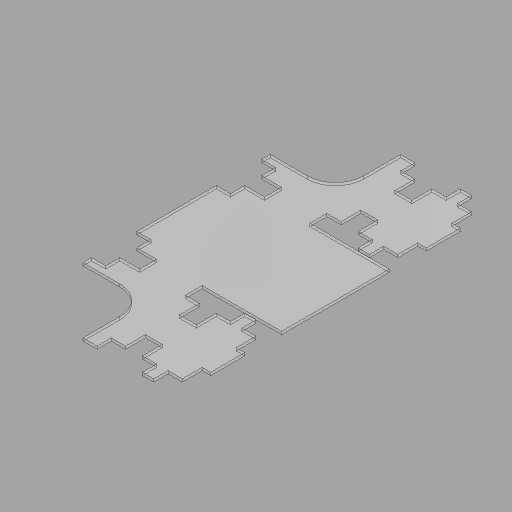
# Autodesk Inventor part: 2024-100-006-Electrical-Plate
Saved by Autodesk Inventor 2024.2 (Build 282272000, 272)
## iProperties
Created: 2024-02-14
Part Number: 2024-100-006-Electrical-Plate
Material: Polycarbonate, Clear
Document SubType Name: Modeling
Designer: rohan
Density: 1.2 g/cm^3
Appearance: Polycarbonate - Clear
Author: rohan
Autodesk Inventor part; units mm, degrees
ref_plane "YZ Plane" through (0, 0, 0) normal (1, 0, 0) x (0, 1, 0)
ref_plane "XZ Plane" through (0, 0, 0) normal (0, 1, 0) x (-1, 0, 0)
ref_plane "XY Plane" through (0, 0, 0) normal (0, 0, 1) x (1, 0, 0)
sketch "Sketch1" plane through (0, 0, 0) normal (0, 1, 0) x (-1, 0, 0)
  line L0 (355.6, 355.6) -> (-355.6, 355.6)
  line L1 (-355.6, 355.6) -> (-355.6, -355.6)
  line L2 (-355.6, -355.6) -> (355.6, -355.6)
  line L3 (355.6, -355.6) -> (355.6, 355.6)
  line L4 (355.6, 355.6) -> (-355.6, -355.6) construction
  line L5 (-355.6, 355.6) -> (355.6, -355.6) construction
  point P0 (0, 0)
  dimension "d0" = 711.2
  dimension "d1" = 711.2
  constraints: 12 end point, 2 midpoint, 2 parallel, 1 horizontal, 1 perpendicular
  measures "d0" distance of L2.end L1.end
  measures "d1" distance of L1.end L0.end
extrude "Extrusion1" add sketch "Sketch1" along normal blind 6.35
sketch "Sketch2" plane through (0, 6.35, 0) normal (0, 1, 0) x (1, 0, 0)
  line L0 (355.6, -355.6) -> (355.6, 355.6) projected
  line L1 (355.6, 355.6) -> (-355.6, 355.6) projected
  line L2 (-355.6, 355.6) -> (-355.6, -355.6) projected
  line L3 (-355.6, -355.6) -> (355.6, -355.6) projected
  line L4 (-355.6, -355.6) -> (-279.4, -355.6)
  line L5 (-279.4, -355.6) -> (-279.4, -323.85)
  line L6 (-279.4, -323.85) -> (-323.85, -323.85)
  line L7 (-323.85, -323.85) -> (-323.85, -279.4)
  line L8 (-323.85, -279.4) -> (-355.6, -279.4)
  line L9 (-355.6, 355.6) -> (-355.6, -355.6) projected
  line L10 (-355.6, -279.4) -> (-355.6, -355.6)
  line L11 (-424.5174, 0) -> (433.8456, 0) construction
  line L12 (0, -429.639) -> (0, 434.6438) construction
  line L13 (-355.6, -355.6) -> (-355.6, 355.6)
  line L14 (-355.6, 355.6) -> (355.6, 355.6)
  line L15 (-279.4, 355.6) -> (-279.4, 323.85)
  line L16 (-279.4, 323.85) -> (-323.85, 323.85)
  line L17 (-323.85, 323.85) -> (-323.85, 279.4)
  line L18 (-323.85, 279.4) -> (-355.6, 279.4)
  line L19 (355.6, 355.6) -> (355.6, -355.6)
  line L20 (355.6, -355.6) -> (279.4, -355.6)
  line L21 (279.4, -355.6) -> (279.4, -323.85)
  line L22 (279.4, -323.85) -> (323.85, -323.85)
  line L23 (323.85, -323.85) -> (323.85, -279.4)
  line L24 (323.85, -279.4) -> (355.6, -279.4)
  line L25 (355.6, 355.6) -> (355.6, -355.6)
  line L26 (355.6, -279.4) -> (355.6, -355.6)
  line L27 (323.85, 279.4) -> (355.6, 279.4)
  line L28 (279.4, 355.6) -> (279.4, 323.85)
  line L29 (279.4, 323.85) -> (323.85, 323.85)
  line L30 (323.85, 323.85) -> (323.85, 279.4)
  line L31 (355.6, -355.6) -> (355.6, 355.6)
  point P0 (0, 0)
  dimension "d4" = 76.2
  dimension "d5" = 31.75
  dimension "d6" = 44.45
  dimension "d7" = 44.45
  constraints: 54 end point, 21 symmetric about line, 6 point on line, 3 perpendicular, 2 vertical, 1 collinear, 1 horizontal
  measures "d4" distance of L2.end L4.end
  measures "d5" distance of L4.end L5.end
  measures "d6" distance of L5.end L6.end
  measures "d7" distance of L6.end L7.end
extrude "Extrusion2" cut sketch "Sketch2" against normal blind 6.35 contours L3 L21 L22 L23 L24 L0 | L27 L30 L29 L28 L1 L0 | L3 L2 L8 L7 L6 L5 | L15 L16 L17 L18 L2 L1
sketch "Sketch3" plane through (0, 6.35, 0) normal (0, 1, 0) x (1, 0, 0)
  line L0 (355.6, 279.4) -> (323.85, 279.4) projected
  line L1 (323.85, 279.4) -> (323.85, 323.85) projected
  line L2 (323.85, 323.85) -> (279.4, 323.85) projected
  line L3 (279.4, 323.85) -> (279.4, 355.6) projected
  line L4 (279.4, 355.6) -> (-279.4, 355.6) projected
  line L5 (-279.4, 355.6) -> (-279.4, 323.85) projected
  line L6 (-279.4, 323.85) -> (-323.85, 323.85) projected
  line L7 (-323.85, 323.85) -> (-323.85, 279.4) projected
  line L8 (-323.85, 279.4) -> (-355.6, 279.4) projected
  line L9 (-355.6, 279.4) -> (-355.6, -279.4) projected
  line L10 (-355.6, -279.4) -> (-323.85, -279.4) projected
  line L11 (-323.85, -279.4) -> (-323.85, -323.85) projected
  line L12 (-323.85, -323.85) -> (-279.4, -323.85) projected
  line L13 (-279.4, -323.85) -> (-279.4, -355.6) projected
  line L14 (-279.4, -355.6) -> (279.4, -355.6) projected
  line L15 (279.4, -355.6) -> (279.4, -323.85) projected
  line L16 (279.4, -323.85) -> (323.85, -323.85) projected
  line L17 (323.85, -323.85) -> (323.85, -279.4) projected
  line L18 (323.85, -279.4) -> (355.6, -279.4) projected
  line L19 (355.6, -279.4) -> (355.6, 279.4) projected
  line L20 (-279.4, -355.6) -> (-355.6, -355.6)
  line L21 (-355.6, -355.6) -> (-355.6, -279.4)
  line L22 (-355.6, -355.6) -> (-355.6, -190.5)
  line L23 (-355.6, 279.4) -> (-355.6, -279.4) projected
  line L24 (-355.6, -190.5) -> (-323.85, -190.5)
  line L25 (-323.85, -190.5) -> (-323.85, -158.75)
  line L26 (-323.85, -158.75) -> (-279.4, -158.75)
  line L27 (-279.4, -158.75) -> (-279.4, -120.65)
  line L28 (-279.4, -120.65) -> (-323.85, -120.65)
  line L29 (-323.85, -120.65) -> (-323.85, -88.9)
  line L30 (-323.85, -88.9) -> (-355.6, -88.9)
  line L31 (-355.6, -88.9) -> (-355.6, -190.5)
  line L32 (-429.9144, 0) -> (459.921, 0) construction
  line L33 (-355.6, -279.4) -> (-355.6, 279.4)
  line L34 (-355.6, 190.5) -> (-323.85, 190.5)
  line L35 (-323.85, 190.5) -> (-323.85, 158.75)
  line L36 (-323.85, 158.75) -> (-279.4, 158.75)
  line L37 (-279.4, 158.75) -> (-279.4, 120.65)
  line L38 (-279.4, 120.65) -> (-323.85, 120.65)
  line L39 (-323.85, 120.65) -> (-323.85, 88.9)
  line L40 (-323.85, 88.9) -> (-355.6, 88.9)
  point P0 (0, 0)
  dimension "d10" = 165.1
  dimension "d11" = 31.75
  dimension "d12" = 31.75
  dimension "d13" = 44.45
  dimension "d14" = 38.1
  dimension "d15" = 31.75
  constraints: 40 end point, 10 symmetric about line, 5 perpendicular, 4 horizontal, 2 point on line, 1 collinear, 1 vertical
  measures "d10" distance of L20.end L22.end
  measures "d11" distance of L22.end L24.end
  measures "d12" distance of L24.end L25.end
  measures "d13" distance of L25.end L26.end
  measures "d14" distance of L26.end L27.end
  measures "d15" distance of L28.end L29.end
extrude "Extrusion3" cut sketch "Sketch3" against normal blind 6.35 contours L9 L30 L29 L28 L27 L26 L25 L24 | L34 L35 L36 L37 L38 L39 L40 L9
sketch "Sketch4" plane through (0, 6.35, 0) normal (0, 1, 0) x (1, 0, 0)
  line L0 (-323.85, 88.9) -> (-355.6, 88.9) projected
  line L1 (-355.6, 88.9) -> (-355.6, -88.9) projected
  line L2 (-355.6, -88.9) -> (-323.85, -88.9) projected
  line L3 (-323.85, -88.9) -> (-323.85, -120.65) projected
  line L4 (-323.85, -120.65) -> (-279.4, -120.65) projected
  line L5 (-279.4, -120.65) -> (-279.4, -158.75) projected
  line L6 (-279.4, -158.75) -> (-323.85, -158.75) projected
  line L7 (-323.85, -158.75) -> (-323.85, -190.5) projected
  line L8 (-323.85, -190.5) -> (-355.6, -190.5) projected
  line L9 (-355.6, -190.5) -> (-355.6, -279.4) projected
  line L10 (-355.6, -279.4) -> (-323.85, -279.4) projected
  line L11 (-323.85, -279.4) -> (-323.85, -323.85) projected
  line L12 (-323.85, -323.85) -> (-279.4, -323.85) projected
  line L13 (-279.4, -323.85) -> (-279.4, -355.6) projected
  line L14 (-279.4, -355.6) -> (279.4, -355.6) projected
  line L15 (279.4, -355.6) -> (279.4, -323.85) projected
  line L16 (279.4, -323.85) -> (323.85, -323.85) projected
  line L17 (323.85, -323.85) -> (323.85, -279.4) projected
  line L18 (323.85, -279.4) -> (355.6, -279.4) projected
  line L19 (355.6, -279.4) -> (355.6, 279.4) projected
  line L20 (355.6, 279.4) -> (323.85, 279.4) projected
  line L21 (323.85, 279.4) -> (323.85, 323.85) projected
  line L22 (323.85, 323.85) -> (279.4, 323.85) projected
  line L23 (279.4, 323.85) -> (279.4, 355.6) projected
  line L24 (279.4, 355.6) -> (-279.4, 355.6) projected
  line L25 (-279.4, 355.6) -> (-279.4, 323.85) projected
  line L26 (-279.4, 323.85) -> (-323.85, 323.85) projected
  line L27 (-323.85, 323.85) -> (-323.85, 279.4) projected
  line L28 (-323.85, 279.4) -> (-355.6, 279.4) projected
  line L29 (-355.6, 279.4) -> (-355.6, 190.5) projected
  line L30 (-355.6, 190.5) -> (-323.85, 190.5) projected
  line L31 (-323.85, 190.5) -> (-323.85, 158.75) projected
  line L32 (-323.85, 158.75) -> (-279.4, 158.75) projected
  line L33 (-279.4, 158.75) -> (-279.4, 120.65) projected
  line L34 (-279.4, 120.65) -> (-323.85, 120.65) projected
  line L35 (-323.85, 120.65) -> (-323.85, 88.9) projected
  line L36 (-279.4, -355.6) -> (-355.6, -355.6)
  line L37 (-355.6, -355.6) -> (-209.55, -355.6)
  line L38 (-209.55, -355.6) -> (-209.55, -273.05)
  line L39 (-273.05, -209.55) -> (-355.6, -209.55)
  line L40 (-355.6, -355.6) -> (-355.6, -209.55)
  arc A0 (-209.55, -273.05) -> (-273.05, -209.55) centre (-273.05, -273.05) ccw
  line L41 (-440.4629, 0) -> (-405.206, 0)
  line L42 (-355.6, 190.5) -> (-355.6, 279.4)
  line L43 (-355.6, 355.6) -> (-209.55, 355.6)
  line L44 (-209.55, 355.6) -> (-209.55, 273.05)
  line L45 (-273.05, 209.55) -> (-355.6, 209.55)
  line L46 (-355.6, 355.6) -> (-355.6, 209.55)
  arc A1 (-273.05, 209.55) -> (-209.55, 273.05) centre (-273.05, 273.05) ccw
  line L47 (0, -524.0203) -> (0, -477.0111)
  line L48 (323.85, 88.9) -> (355.6, 88.9)
  line L49 (355.6, 88.9) -> (355.6, -88.9)
  line L50 (355.6, -88.9) -> (323.85, -88.9)
  line L51 (323.85, -88.9) -> (323.85, -120.65)
  line L52 (323.85, -120.65) -> (279.4, -120.65)
  line L53 (279.4, -120.65) -> (279.4, -158.75)
  line L54 (279.4, -158.75) -> (323.85, -158.75)
  line L55 (323.85, -158.75) -> (323.85, -190.5)
  line L56 (323.85, -190.5) -> (355.6, -190.5)
  line L57 (355.6, -190.5) -> (355.6, -279.4)
  line L58 (355.6, -279.4) -> (323.85, -279.4)
  line L59 (323.85, -279.4) -> (323.85, -323.85)
  line L60 (323.85, -323.85) -> (279.4, -323.85)
  line L61 (279.4, -323.85) -> (279.4, -355.6)
  line L62 (279.4, 355.6) -> (279.4, 323.85)
  line L63 (279.4, 323.85) -> (323.85, 323.85)
  line L64 (323.85, 323.85) -> (323.85, 279.4)
  line L65 (323.85, 279.4) -> (355.6, 279.4)
  line L66 (355.6, 279.4) -> (355.6, 190.5)
  line L67 (355.6, 190.5) -> (323.85, 190.5)
  line L68 (323.85, 190.5) -> (323.85, 158.75)
  line L69 (323.85, 158.75) -> (279.4, 158.75)
  line L70 (279.4, 158.75) -> (279.4, 120.65)
  line L71 (279.4, 120.65) -> (323.85, 120.65)
  line L72 (323.85, 120.65) -> (323.85, 88.9)
  line L73 (279.4, -355.6) -> (355.6, -355.6)
  line L74 (355.6, -355.6) -> (209.55, -355.6)
  line L75 (209.55, -355.6) -> (209.55, -273.05)
  line L76 (273.05, -209.55) -> (355.6, -209.55)
  line L77 (355.6, -355.6) -> (355.6, -209.55)
  arc A2 (273.05, -209.55) -> (209.55, -273.05) centre (273.05, -273.05) ccw
  line L78 (273.05, 209.55) -> (355.6, 209.55)
  arc A3 (209.55, 273.05) -> (273.05, 209.55) centre (273.05, 273.05) ccw
  line L79 (355.6, 190.5) -> (355.6, 279.4)
  line L80 (355.6, 355.6) -> (355.6, 209.55)
  line L81 (355.6, 355.6) -> (209.55, 355.6)
  line L82 (209.55, 355.6) -> (209.55, 273.05)
  point P0 (0, 0)
  point P1 (-209.55, -209.55)
  point P2 (209.55, -209.55)
  point P3 (-209.55, 355.6)
  point P4 (209.55, 355.6)
  point P5 (209.55, -355.6)
  dimension "d18" = 146.05
  dimension "d19" = 146.05
  dimension "d20" = 63.5
  constraints: 94 end point, 35 symmetric about line, 9 point on line, 8 point on circle, 4 centre point, 2 horizontal, 2 perpendicular, 2 tangent, 1 collinear, 1 vertical, 3 other
  measures "d18" distance of L36.end L37.end
  measures "d19" distance of L37.end point (-209.55, -209.55)
  measures "d20" radius of A0
extrude "Extrusion4" cut sketch "Sketch4" against normal blind 6.35 contours L29 L28 L27 L26 L25 L24 L44 A1 L45 | L46 L43 L25 L26 L27 L28 | L39 A0 L38 L14 L13 L12 L11 L10 L9 | L10 L11 L12 L13 L36 L40 | L24 L23 L22 L21 L20 L19 L78 A3 L82 | L81 L80 L20 L21 L22 L23 | L75 A2 L76 L19 L18 L17 L16 L15 L14 | L15 L16 L17 L18 L77 L73
sketch "Sketch5" plane through (0, 6.35, 0) normal (0, 1, 0) x (1, 0, 0)
  line L0 (-209.55, 355.6) -> (-209.55, 273.05) projected
  arc A0 (-273.05, 209.55) -> (-209.55, 273.05) centre (-273.05, 273.05) ccw projected
  line L1 (-273.05, 209.55) -> (-355.6, 209.55) projected
  line L2 (-355.6, 209.55) -> (-355.6, 190.5) projected
  line L3 (-355.6, 190.5) -> (-323.85, 190.5) projected
  line L4 (-323.85, 190.5) -> (-323.85, 158.75) projected
  line L5 (-323.85, 158.75) -> (-279.4, 158.75) projected
  line L6 (-279.4, 158.75) -> (-279.4, 120.65) projected
  line L7 (-279.4, 120.65) -> (-323.85, 120.65) projected
  line L8 (-323.85, 120.65) -> (-323.85, 88.9) projected
  line L9 (-323.85, 88.9) -> (-355.6, 88.9) projected
  line L10 (-355.6, 88.9) -> (-355.6, -88.9) projected
  line L11 (-355.6, -88.9) -> (-323.85, -88.9) projected
  line L12 (-323.85, -88.9) -> (-323.85, -120.65) projected
  line L13 (-323.85, -120.65) -> (-279.4, -120.65) projected
  line L14 (-279.4, -120.65) -> (-279.4, -158.75) projected
  line L15 (-279.4, -158.75) -> (-323.85, -158.75) projected
  line L16 (-323.85, -158.75) -> (-323.85, -190.5) projected
  line L17 (-323.85, -190.5) -> (-355.6, -190.5) projected
  line L18 (-355.6, -190.5) -> (-355.6, -209.55) projected
  line L19 (-355.6, -209.55) -> (-273.05, -209.55) projected
  arc A1 (-209.55, -273.05) -> (-273.05, -209.55) centre (-273.05, -273.05) ccw projected
  line L20 (-209.55, -273.05) -> (-209.55, -355.6) projected
  line L21 (-209.55, -355.6) -> (209.55, -355.6) projected
  line L22 (209.55, -355.6) -> (209.55, -273.05) projected
  arc A2 (273.05, -209.55) -> (209.55, -273.05) centre (273.05, -273.05) ccw projected
  line L23 (273.05, -209.55) -> (355.6, -209.55) projected
  line L24 (355.6, -209.55) -> (355.6, 209.55) projected
  line L25 (355.6, 209.55) -> (273.05, 209.55) projected
  arc A3 (209.55, 273.05) -> (273.05, 209.55) centre (273.05, 273.05) ccw projected
  line L26 (209.55, 273.05) -> (209.55, 355.6) projected
  line L27 (209.55, 355.6) -> (-209.55, 355.6) projected
  line L28 (-355.6, -209.55) -> (-355.6, -355.6)
  line L29 (-355.6, -355.6) -> (-196.85, -355.6)
  line L30 (-209.55, -355.6) -> (209.55, -355.6) projected
  line L31 (-196.85, -355.6) -> (-228.6, -355.6)
  line L32 (-196.85, -355.6) -> (-196.85, -323.85)
  line L33 (-196.85, -323.85) -> (-170.18, -323.85)
  line L34 (-167.5384, -321.2084) -> (-170.18, -323.85)
  line L35 (-167.5384, -321.2084) -> (-167.5384, -283.1084)
  line L36 (-157.48, -273.05) -> (-167.5384, -283.1084)
  line L37 (-157.48, -273.05) -> (-114.1222, -273.05)
  line L38 (-135.8011, -273.05) -> (-135.8011, -278.0792)
  line L39 (-104.0638, -321.2084) -> (-104.0638, -283.1084)
  line L40 (-114.1222, -273.05) -> (-104.0638, -283.1084)
  line L41 (-104.0638, -321.2084) -> (-101.4222, -323.85)
  line L42 (-101.4222, -323.85) -> (-79.9338, -323.85)
  line L43 (-79.9338, -323.85) -> (-79.9338, -355.6)
  line L44 (-488.7468, 0) -> (-430.53, 0)
  line L45 (-196.85, 355.6) -> (-196.85, 323.85)
  line L46 (-196.85, 323.85) -> (-170.18, 323.85)
  line L47 (-167.5384, 321.2084) -> (-170.18, 323.85)
  line L48 (-167.5384, 321.2084) -> (-167.5384, 283.1084)
  line L49 (-157.48, 273.05) -> (-167.5384, 283.1084)
  line L50 (-157.48, 273.05) -> (-114.1222, 273.05)
  line L51 (-135.8011, 273.05) -> (-135.8011, 278.0792)
  line L52 (-114.1222, 273.05) -> (-104.0638, 283.1084)
  line L53 (-104.0638, 321.2084) -> (-104.0638, 283.1084)
  line L54 (-104.0638, 321.2084) -> (-101.4222, 323.85)
  line L55 (-101.4222, 323.85) -> (-79.9338, 323.85)
  line L56 (-79.9338, 323.85) -> (-79.9338, 355.6)
  line L57 (0, -550.9534) -> (0, -488.7468)
  line L58 (209.55, 355.6) -> (209.55, 273.05)
  line L59 (196.85, -355.6) -> (196.85, -323.85)
  line L60 (196.85, -323.85) -> (170.18, -323.85)
  line L61 (167.5384, -321.2084) -> (170.18, -323.85)
  line L62 (167.5384, -321.2084) -> (167.5384, -283.1084)
  line L63 (157.48, -273.05) -> (167.5384, -283.1084)
  line L64 (157.48, -273.05) -> (114.1222, -273.05)
  line L65 (135.8011, -273.05) -> (135.8011, -278.0792)
  line L66 (114.1222, -273.05) -> (104.0638, -283.1084)
  line L67 (104.0638, -321.2084) -> (104.0638, -283.1084)
  line L68 (104.0638, -321.2084) -> (101.4222, -323.85)
  line L69 (101.4222, -323.85) -> (79.9338, -323.85)
  line L70 (79.9338, -323.85) -> (79.9338, -355.6)
  line L71 (79.9338, 323.85) -> (79.9338, 355.6)
  line L72 (101.4222, 323.85) -> (79.9338, 323.85)
  line L73 (104.0638, 321.2084) -> (104.0638, 283.1084)
  line L74 (104.0638, 321.2084) -> (101.4222, 323.85)
  line L75 (114.1222, 273.05) -> (104.0638, 283.1084)
  line L76 (157.48, 273.05) -> (114.1222, 273.05)
  line L77 (157.48, 273.05) -> (167.5384, 283.1084)
  line L78 (167.5384, 321.2084) -> (167.5384, 283.1084)
  line L79 (196.85, 355.6) -> (196.85, 323.85)
  line L80 (196.85, 323.85) -> (170.18, 323.85)
  line L81 (167.5384, 321.2084) -> (170.18, 323.85)
  point P0 (0, 0)
  dimension "d24" = 158.75
  dimension "d25" = 31.75
  dimension "d26" = 31.75
  dimension "d27" = 26.67
  dimension "d30" = 38.1
  dimension "d33" = 43.3578
  dimension "d34" = 21.4884
  constraints: 106 end point, 43 symmetric about line, 4 vertical, 3 horizontal, 3 perpendicular, 3 point on line, 1 midpoint
  measures "d24" distance of L28.end L29.end
  measures "d25" distance of L29.end L31.end
  measures "d26" distance of L29.end L32.end
  measures "d27" distance of L32.end L33.end
  measures "d30" distance of L34.start L35.end
  measures "d33" distance of L36.start L37.end
  measures "d34" distance of L41.end L42.end
extrude "Extrusion5" cut sketch "Sketch5" against normal blind 576.2625 contours L27 L79 L80 L81 L78 L77 L76 L75 L73 L74 L72 L71 | L21 L70 L69 L68 L67 L66 L64 L63 L62 L61 L60 L59
sketch "Sketch6" plane through (0, 6.35, 0) normal (0, 1, 0) x (1, 0, 0)
  line L0 (-279.4, 158.75) -> (-279.4, 120.65) projected
  line L1 (-279.4, -120.65) -> (-279.4, -158.75) projected
  line L2 (-111.125, 158.75) -> (-111.125, 120.65)
  line L3 (-323.85, 120.65) -> (-279.4, 120.65) projected
  line L4 (196.85, 355.6) -> (196.85, 323.85) projected
  line L5 (196.85, 323.85) -> (170.18, 323.85) projected
  line L6 (170.18, 323.85) -> (167.5384, 321.2084) projected
  line L7 (167.5384, 321.2084) -> (167.5384, 283.1084) projected
  line L8 (167.5384, 283.1084) -> (157.48, 273.05) projected
  line L9 (157.48, 273.05) -> (114.1222, 273.05) projected
  line L10 (114.1222, 273.05) -> (104.0638, 283.1084) projected
  line L11 (104.0638, 283.1084) -> (104.0638, 321.2084) projected
  line L12 (104.0638, 321.2084) -> (101.4222, 323.85) projected
  line L13 (101.4222, 323.85) -> (79.9338, 323.85) projected
  line L14 (79.9338, 323.85) -> (79.9338, 355.6) projected
  line L15 (79.9338, 355.6) -> (-209.55, 355.6) projected
  line L16 (-209.55, 355.6) -> (-209.55, 273.05) projected
  arc A0 (-273.05, 209.55) -> (-209.55, 273.05) centre (-273.05, 273.05) ccw projected
  line L17 (-273.05, 209.55) -> (-355.6, 209.55) projected
  line L18 (-355.6, 209.55) -> (-355.6, 190.5) projected
  line L19 (-355.6, 190.5) -> (-323.85, 190.5) projected
  line L20 (-323.85, 190.5) -> (-323.85, 158.75) projected
  line L21 (-323.85, 158.75) -> (-279.4, 158.75) projected
  line L22 (-279.4, 158.75) -> (-279.4, 120.65) projected
  line L23 (-279.4, 120.65) -> (-323.85, 120.65) projected
  line L24 (-323.85, 120.65) -> (-323.85, 88.9) projected
  line L25 (-323.85, 88.9) -> (-355.6, 88.9) projected
  line L26 (-355.6, 88.9) -> (-355.6, -88.9) projected
  line L27 (-355.6, -88.9) -> (-323.85, -88.9) projected
  line L28 (-323.85, -88.9) -> (-323.85, -120.65) projected
  line L29 (-323.85, -120.65) -> (-279.4, -120.65) projected
  line L30 (-279.4, -120.65) -> (-279.4, -158.75) projected
  line L31 (-279.4, -158.75) -> (-323.85, -158.75) projected
  line L32 (-323.85, -158.75) -> (-323.85, -190.5) projected
  line L33 (-323.85, -190.5) -> (-355.6, -190.5) projected
  line L34 (-355.6, -190.5) -> (-355.6, -209.55) projected
  line L35 (-355.6, -209.55) -> (-273.05, -209.55) projected
  arc A1 (-209.55, -273.05) -> (-273.05, -209.55) centre (-273.05, -273.05) ccw projected
  line L36 (-209.55, -273.05) -> (-209.55, -355.6) projected
  line L37 (-209.55, -355.6) -> (79.9338, -355.6) projected
  line L38 (79.9338, -355.6) -> (79.9338, -323.85) projected
  line L39 (79.9338, -323.85) -> (101.4222, -323.85) projected
  line L40 (101.4222, -323.85) -> (104.0638, -321.2084) projected
  line L41 (104.0638, -321.2084) -> (104.0638, -283.1084) projected
  line L42 (104.0638, -283.1084) -> (114.1222, -273.05) projected
  line L43 (114.1222, -273.05) -> (157.48, -273.05) projected
  line L44 (157.48, -273.05) -> (167.5384, -283.1084) projected
  line L45 (167.5384, -283.1084) -> (167.5384, -321.2084) projected
  line L46 (167.5384, -321.2084) -> (170.18, -323.85) projected
  line L47 (170.18, -323.85) -> (196.85, -323.85) projected
  line L48 (196.85, -323.85) -> (196.85, -355.6) projected
  line L49 (196.85, -355.6) -> (209.55, -355.6) projected
  line L50 (209.55, -355.6) -> (209.55, -273.05) projected
  arc A2 (273.05, -209.55) -> (209.55, -273.05) centre (273.05, -273.05) ccw projected
  line L51 (273.05, -209.55) -> (355.6, -209.55) projected
  line L52 (355.6, -209.55) -> (355.6, 209.55) projected
  line L53 (355.6, 209.55) -> (273.05, 209.55) projected
  arc A3 (209.55, 273.05) -> (273.05, 209.55) centre (273.05, 273.05) ccw projected
  line L54 (209.55, 273.05) -> (209.55, 355.6) projected
  line L55 (209.55, 355.6) -> (196.85, 355.6) projected
  line L56 (101.6, 120.65) -> (57.15, 120.65)
  line L57 (104.0638, 190.5) -> (101.6, 190.5)
  line L58 (101.6, 190.5) -> (101.6, 158.75)
  line L59 (101.6, 158.75) -> (57.15, 158.75)
  line L60 (101.6, 120.65) -> (101.6, 88.9)
  line L61 (101.6, 88.9) -> (104.0638, 88.9)
  line L62 (142.1384, 190.5) -> (142.1384, 88.9)
  line L63 (142.1384, 88.9) -> (133.35, 88.9)
  line L64 (101.6, 190.5) -> (101.6, 196.85)
  line L65 (101.6, 196.85) -> (142.1384, 196.85)
  line L66 (142.1384, 196.85) -> (142.1384, 190.5)
  line L67 (142.1384, 88.9) -> (142.1384, 82.55)
  line L68 (142.1384, 82.55) -> (101.6, 82.55)
  line L69 (101.6, 82.55) -> (101.6, 88.9)
  line L70 (57.15, 158.75) -> (44.45, 158.75)
  line L71 (44.45, 158.75) -> (44.45, 120.65)
  line L72 (44.45, 120.65) -> (57.15, 120.65)
  line L73 (396.3517, 0) -> (373.7228, 0)
  line L74 (101.6, -88.9) -> (104.0638, -88.9)
  line L75 (101.6, -120.65) -> (101.6, -88.9)
  line L76 (101.6, -120.65) -> (57.15, -120.65)
  line L77 (101.6, -158.75) -> (57.15, -158.75)
  line L78 (101.6, -190.5) -> (101.6, -158.75)
  line L79 (104.0638, -190.5) -> (101.6, -190.5)
  line L80 (142.1384, -190.5) -> (142.1384, -88.9)
  line L81 (142.1384, -88.9) -> (133.35, -88.9)
  line L82 (101.6, -190.5) -> (101.6, -196.85)
  line L83 (101.6, -196.85) -> (142.1384, -196.85)
  line L84 (142.1384, -196.85) -> (142.1384, -190.5)
  line L85 (142.1384, -88.9) -> (142.1384, -82.55)
  line L86 (142.1384, -82.55) -> (101.6, -82.55)
  line L87 (101.6, -82.55) -> (101.6, -88.9)
  line L88 (57.15, -158.75) -> (44.45, -158.75)
  line L89 (44.45, -158.75) -> (44.45, -120.65)
  line L90 (44.45, -120.65) -> (57.15, -120.65)
  point P0 (0, 0)
  point P1 (-111.125, 139.7)
  point P2 (-279.4, 139.7)
  dimension "d38" = 168.275
  dimension "d42" = 6.35
  dimension "d43" = 6.35
  dimension "d44" = 12.7
  constraints: 72 end point, 28 symmetric about line, 6 perpendicular, 6 point on line, 2 horizontal, 2 midpoint, 2 vertical, 1 collinear
  measures "d38" distance between parallel lines of L2 L0
  measures "d42" distance of L58.start L64.end
  measures "d43" distance of L62.end L67.end
  measures "d44" distance of L59.end L70.end
extrude "Extrusion6" cut sketch "Sketch6" against normal blind 365.125 contours L56 L72 L71 L70 L59 L58 L64 L65 L66 L62 L67 L68 L69 L60 | L75 L87 L86 L85 L80 L84 L83 L82 L78 L77 L88 L89 L90 L76
sketch "Sketch7" plane through (0, 6.35, 0) normal (0, 1, 0) x (1, 0, 0)
  line L0 (142.1384, -82.55) -> (142.1384, -196.85) projected
  line L1 (142.1384, -196.85) -> (101.6, -196.85) projected
  line L2 (101.6, -196.85) -> (101.6, -158.75) projected
  line L3 (101.6, -158.75) -> (44.45, -158.75) projected
  line L4 (44.45, -158.75) -> (44.45, -120.65) projected
  line L5 (44.45, -120.65) -> (101.6, -120.65) projected
  line L6 (101.6, -120.65) -> (101.6, -82.55) projected
  line L7 (101.6, -82.55) -> (142.1384, -82.55) projected
  line L8 (44.45, 158.75) -> (101.6, 158.75) projected
  line L9 (101.6, 158.75) -> (101.6, 196.85) projected
  line L10 (101.6, 196.85) -> (142.1384, 196.85) projected
  line L11 (142.1384, 196.85) -> (142.1384, 82.55) projected
  line L12 (142.1384, 82.55) -> (101.6, 82.55) projected
  line L13 (101.6, 82.55) -> (101.6, 120.65) projected
  line L14 (101.6, 120.65) -> (44.45, 120.65) projected
  line L15 (44.45, 120.65) -> (44.45, 158.75) projected
  line L16 (196.85, 355.6) -> (196.85, 323.85) projected
  line L17 (196.85, 323.85) -> (170.18, 323.85) projected
  line L18 (170.18, 323.85) -> (167.5384, 321.2084) projected
  line L19 (167.5384, 321.2084) -> (167.5384, 283.1084) projected
  line L20 (167.5384, 283.1084) -> (157.48, 273.05) projected
  line L21 (157.48, 273.05) -> (114.1222, 273.05) projected
  line L22 (114.1222, 273.05) -> (104.0638, 283.1084) projected
  line L23 (104.0638, 283.1084) -> (104.0638, 321.2084) projected
  line L24 (104.0638, 321.2084) -> (101.4222, 323.85) projected
  line L25 (101.4222, 323.85) -> (79.9338, 323.85) projected
  line L26 (79.9338, 323.85) -> (79.9338, 355.6) projected
  line L27 (79.9338, 355.6) -> (-209.55, 355.6) projected
  line L28 (-209.55, 355.6) -> (-209.55, 273.05) projected
  arc A0 (-273.05, 209.55) -> (-209.55, 273.05) centre (-273.05, 273.05) ccw projected
  line L29 (-273.05, 209.55) -> (-355.6, 209.55) projected
  line L30 (-355.6, 209.55) -> (-355.6, 190.5) projected
  line L31 (-355.6, 190.5) -> (-323.85, 190.5) projected
  line L32 (-323.85, 190.5) -> (-323.85, 158.75) projected
  line L33 (-323.85, 158.75) -> (-279.4, 158.75) projected
  line L34 (-279.4, 158.75) -> (-279.4, 120.65) projected
  line L35 (-279.4, 120.65) -> (-323.85, 120.65) projected
  line L36 (-323.85, 120.65) -> (-323.85, 88.9) projected
  line L37 (-323.85, 88.9) -> (-355.6, 88.9) projected
  line L38 (-355.6, 88.9) -> (-355.6, -88.9) projected
  line L39 (-355.6, -88.9) -> (-323.85, -88.9) projected
  line L40 (-323.85, -88.9) -> (-323.85, -120.65) projected
  line L41 (-323.85, -120.65) -> (-279.4, -120.65) projected
  line L42 (-279.4, -120.65) -> (-279.4, -158.75) projected
  line L43 (-279.4, -158.75) -> (-323.85, -158.75) projected
  line L44 (-323.85, -158.75) -> (-323.85, -190.5) projected
  line L45 (-323.85, -190.5) -> (-355.6, -190.5) projected
  line L46 (-355.6, -190.5) -> (-355.6, -209.55) projected
  line L47 (-355.6, -209.55) -> (-273.05, -209.55) projected
  arc A1 (-209.55, -273.05) -> (-273.05, -209.55) centre (-273.05, -273.05) ccw projected
  line L48 (-209.55, -273.05) -> (-209.55, -355.6) projected
  line L49 (-209.55, -355.6) -> (79.9338, -355.6) projected
  line L50 (79.9338, -355.6) -> (79.9338, -323.85) projected
  line L51 (79.9338, -323.85) -> (101.4222, -323.85) projected
  line L52 (101.4222, -323.85) -> (104.0638, -321.2084) projected
  line L53 (104.0638, -321.2084) -> (104.0638, -283.1084) projected
  line L54 (104.0638, -283.1084) -> (114.1222, -273.05) projected
  line L55 (114.1222, -273.05) -> (157.48, -273.05) projected
  line L56 (157.48, -273.05) -> (167.5384, -283.1084) projected
  line L57 (167.5384, -283.1084) -> (167.5384, -321.2084) projected
  line L58 (167.5384, -321.2084) -> (170.18, -323.85) projected
  line L59 (170.18, -323.85) -> (196.85, -323.85) projected
  line L60 (196.85, -323.85) -> (196.85, -355.6) projected
  line L61 (196.85, -355.6) -> (209.55, -355.6) projected
  line L62 (209.55, -355.6) -> (209.55, -273.05) projected
  arc A2 (273.05, -209.55) -> (209.55, -273.05) centre (273.05, -273.05) ccw projected
  line L63 (273.05, -209.55) -> (355.6, -209.55) projected
  line L64 (355.6, -209.55) -> (355.6, 209.55) projected
  line L65 (355.6, 209.55) -> (273.05, 209.55) projected
  arc A3 (209.55, 273.05) -> (273.05, 209.55) centre (273.05, 273.05) ccw projected
  line L66 (209.55, 273.05) -> (209.55, 355.6) projected
  line L67 (209.55, 355.6) -> (196.85, 355.6) projected
  line L68 (50.8, -355.6) -> (50.8, -323.85)
  line L69 (50.8, -323.85) -> (19.05, -323.85)
  line L70 (19.05, -323.85) -> (19.05, -279.4)
  line L71 (19.05, -279.4) -> (-19.05, -279.4)
  line L72 (-19.05, -279.4) -> (-19.05, -323.85)
  line L73 (-19.05, -323.85) -> (-50.8, -323.85)
  line L74 (-50.8, -323.85) -> (-50.8, -355.6)
  line L75 (-63.5, -355.6) -> (-63.5, -342.9)
  line L76 (-177.8, -355.6) -> (-177.8, -323.85)
  line L77 (-177.8, -323.85) -> (-146.05, -323.85)
  line L78 (-146.05, -323.85) -> (-146.05, -279.4)
  line L79 (-146.05, -279.4) -> (-107.95, -279.4)
  line L80 (-107.95, -279.4) -> (-107.95, -323.85)
  line L81 (-107.95, -323.85) -> (-76.2, -323.85)
  line L82 (-76.2, -323.85) -> (-76.2, -355.6)
  line L83 (402.714, 0) -> (463.6006, 0)
  line L84 (50.8, 355.6) -> (50.8, 323.85)
  line L85 (50.8, 323.85) -> (19.05, 323.85)
  line L86 (19.05, 323.85) -> (19.05, 279.4)
  line L87 (19.05, 279.4) -> (-19.05, 279.4)
  line L88 (-19.05, 279.4) -> (-19.05, 323.85)
  line L89 (-19.05, 323.85) -> (-50.8, 323.85)
  line L90 (-50.8, 323.85) -> (-50.8, 355.6)
  line L91 (-63.5, 355.6) -> (-63.5, 342.9)
  line L92 (-76.2, 323.85) -> (-76.2, 355.6)
  line L93 (-107.95, 323.85) -> (-76.2, 323.85)
  line L94 (-107.95, 279.4) -> (-107.95, 323.85)
  line L95 (-146.05, 279.4) -> (-107.95, 279.4)
  line L96 (-177.8, 323.85) -> (-146.05, 323.85)
  line L97 (-177.8, 355.6) -> (-177.8, 323.85)
  line L98 (-146.05, 323.85) -> (-146.05, 279.4)
  line L99 (-146.05, -241.3) -> (-70.7106, -241.3)
  line L100 (50.8, -127) -> (50.8, -158.75)
  line L101 (50.8, -158.75) -> (19.05, -158.75)
  line L102 (19.05, -158.75) -> (19.05, -203.2)
  line L103 (19.05, -203.2) -> (-19.05, -203.2)
  line L104 (-19.05, -203.2) -> (-19.05, -158.75)
  line L105 (-19.05, -158.75) -> (-50.8, -158.75)
  line L106 (-50.8, -158.75) -> (-50.8, -127)
  line L107 (-63.5, -127) -> (-63.5, -139.7)
  line L108 (-76.2, -158.75) -> (-76.2, -127)
  line L109 (-107.95, -158.75) -> (-76.2, -158.75)
  line L110 (-107.95, -203.2) -> (-107.95, -158.75)
  line L111 (-146.05, -203.2) -> (-107.95, -203.2)
  line L112 (-177.8, -158.75) -> (-146.05, -158.75)
  line L113 (-177.8, -127) -> (-177.8, -158.75)
  line L114 (-146.05, -158.75) -> (-146.05, -203.2)
  line L115 (-177.8, -127) -> (-76.2, -127)
  line L116 (-50.8, -127) -> (50.8, -127)
  line L117 (44.45, 158.75) -> (44.45, 120.65)
  line L118 (-63.5, 127) -> (-63.5, 139.7)
  line L119 (-76.2, 158.75) -> (-76.2, 127)
  line L120 (-107.95, 203.2) -> (-107.95, 158.75)
  line L121 (-107.95, 158.75) -> (-76.2, 158.75)
  line L122 (-146.05, 203.2) -> (-107.95, 203.2)
  line L123 (-146.05, 158.75) -> (-146.05, 203.2)
  line L124 (-177.8, 158.75) -> (-146.05, 158.75)
  line L125 (-177.8, 127) -> (-177.8, 158.75)
  line L126 (50.8, 127) -> (50.8, 158.75)
  line L127 (-50.8, 158.75) -> (-50.8, 127)
  line L128 (19.05, 158.75) -> (19.05, 203.2)
  line L129 (19.05, 203.2) -> (-19.05, 203.2)
  line L130 (-19.05, 203.2) -> (-19.05, 158.75)
  line L131 (-19.05, 158.75) -> (-50.8, 158.75)
  line L132 (50.8, 158.75) -> (19.05, 158.75)
  line L133 (-177.8, 127) -> (-76.2, 127)
  line L134 (-50.8, 127) -> (50.8, 127)
  point P0 (0, 0)
  point P1 (-63.5, -349.25)
  point P2 (-127, -279.4)
  point P3 (-127, -203.2)
  point P4 (-127, 203.2)
  dimension "d45" = 31.75
  dimension "d46" = 29.1338
  dimension "d47" = 31.75
  dimension "d48" = 44.45
  dimension "d49" = 38.1
  dimension "d50" = 44.45
  dimension "d51" = 31.75
  dimension "d52" = 12.7
  dimension "d53" = 12.7
  dimension "d56" = 38.1
  constraints: 134 end point, 64 symmetric about line, 5 horizontal, 4 perpendicular, 3 point on line, 2 midpoint, 2 vertical
  measures "d45" distance of L68.start L68.end
  measures "d46" distance between parallel lines of L68 L50
  measures "d47" distance of L68.end L69.end
  measures "d48" distance of L69.end L70.end
  measures "d49" distance of L70.end L71.end
  measures "d50" distance of L71.end L72.end
  measures "d51" distance of L72.end L73.end
  measures "d52" distance of L75.start L75.end
  measures "d53" distance from line of point (-63.5, -349.25) L74
  measures "d56" distance from line of L99 point (-127, -279.4)
extrude "Extrusion7" cut sketch "Sketch7" against normal blind 365.125 contours L3 L4 L116 L100 | L4 L101 L102 L103 L104 L105 L106 L116 | L8 L126 L134 L15 | L15 L134 L127 L131 L130 L129 L128 L132 | L84 L85 L86 L87 L88 L89 L90 L27 | L92 L93 L94 L95 L98 L96 L97 L27 | L49 L74 L73 L72 L71 L70 L69 L68 | L49 L76 L77 L78 L79 L80 L81 L82 | L109 L110 L111 L114 L112 L113 L115 L108 | L119 L133 L125 L124 L123 L122 L120 L121
sketch "Sketch8" plane through (0, 6.35, 0) normal (0, 1, 0) x (1, 0, 0)
  line L0 (101.6, -158.75) -> (19.05, -158.75) projected
  line L1 (19.05, -158.75) -> (19.05, -203.2) projected
  line L2 (19.05, -203.2) -> (-19.05, -203.2) projected
  line L3 (-19.05, -203.2) -> (-19.05, -158.75) projected
  line L4 (-19.05, -158.75) -> (-50.8, -158.75) projected
  line L5 (-50.8, -158.75) -> (-50.8, -127) projected
  line L6 (-50.8, -127) -> (44.45, -127) projected
  line L7 (44.45, -127) -> (44.45, -120.65) projected
  line L8 (44.45, -120.65) -> (101.6, -120.65) projected
  line L9 (101.6, -120.65) -> (101.6, -82.55) projected
  line L10 (101.6, -82.55) -> (142.1384, -82.55) projected
  line L11 (142.1384, -82.55) -> (142.1384, -196.85) projected
  line L12 (142.1384, -196.85) -> (101.6, -196.85) projected
  line L13 (101.6, -196.85) -> (101.6, -158.75) projected
  line L14 (-146.05, -203.2) -> (-146.05, -158.75) projected
  line L15 (-146.05, -158.75) -> (-177.8, -158.75) projected
  line L16 (-177.8, -158.75) -> (-177.8, -127) projected
  line L17 (-177.8, -127) -> (-76.2, -127) projected
  line L18 (-76.2, -127) -> (-76.2, -158.75) projected
  line L19 (-76.2, -158.75) -> (-107.95, -158.75) projected
  line L20 (-107.95, -158.75) -> (-107.95, -203.2) projected
  line L21 (-107.95, -203.2) -> (-146.05, -203.2) projected
  line L22 (-107.95, 158.75) -> (-76.2, 158.75) projected
  line L23 (-76.2, 158.75) -> (-76.2, 127) projected
  line L24 (-76.2, 127) -> (-177.8, 127) projected
  line L25 (-177.8, 127) -> (-177.8, 158.75) projected
  line L26 (-177.8, 158.75) -> (-146.05, 158.75) projected
  line L27 (-146.05, 158.75) -> (-146.05, 203.2) projected
  line L28 (-146.05, 203.2) -> (-107.95, 203.2) projected
  line L29 (-107.95, 203.2) -> (-107.95, 158.75) projected
  line L30 (19.05, 158.75) -> (101.6, 158.75) projected
  line L31 (101.6, 158.75) -> (101.6, 196.85) projected
  line L32 (101.6, 196.85) -> (142.1384, 196.85) projected
  line L33 (142.1384, 196.85) -> (142.1384, 82.55) projected
  line L34 (142.1384, 82.55) -> (101.6, 82.55) projected
  line L35 (101.6, 82.55) -> (101.6, 120.65) projected
  line L36 (101.6, 120.65) -> (44.45, 120.65) projected
  line L37 (44.45, 120.65) -> (44.45, 127) projected
  line L38 (44.45, 127) -> (-50.8, 127) projected
  line L39 (-50.8, 127) -> (-50.8, 158.75) projected
  line L40 (-50.8, 158.75) -> (-19.05, 158.75) projected
  line L41 (-19.05, 158.75) -> (-19.05, 203.2) projected
  line L42 (-19.05, 203.2) -> (19.05, 203.2) projected
  line L43 (19.05, 203.2) -> (19.05, 158.75) projected
  line L44 (-177.8, 323.85) -> (-177.8, 355.6) projected
  line L45 (-177.8, 355.6) -> (-209.55, 355.6) projected
  line L46 (-209.55, 355.6) -> (-209.55, 273.05) projected
  arc A0 (-273.05, 209.55) -> (-209.55, 273.05) centre (-273.05, 273.05) ccw projected
  line L47 (-273.05, 209.55) -> (-355.6, 209.55) projected
  line L48 (-355.6, 209.55) -> (-355.6, 190.5) projected
  line L49 (-355.6, 190.5) -> (-323.85, 190.5) projected
  line L50 (-323.85, 190.5) -> (-323.85, 158.75) projected
  line L51 (-323.85, 158.75) -> (-279.4, 158.75) projected
  line L52 (-279.4, 158.75) -> (-279.4, 120.65) projected
  line L53 (-279.4, 120.65) -> (-323.85, 120.65) projected
  line L54 (-323.85, 120.65) -> (-323.85, 88.9) projected
  line L55 (-323.85, 88.9) -> (-355.6, 88.9) projected
  line L56 (-355.6, 88.9) -> (-355.6, -88.9) projected
  line L57 (-355.6, -88.9) -> (-323.85, -88.9) projected
  line L58 (-323.85, -88.9) -> (-323.85, -120.65) projected
  line L59 (-323.85, -120.65) -> (-279.4, -120.65) projected
  line L60 (-279.4, -120.65) -> (-279.4, -158.75) projected
  line L61 (-279.4, -158.75) -> (-323.85, -158.75) projected
  line L62 (-323.85, -158.75) -> (-323.85, -190.5) projected
  line L63 (-323.85, -190.5) -> (-355.6, -190.5) projected
  line L64 (-355.6, -190.5) -> (-355.6, -209.55) projected
  line L65 (-355.6, -209.55) -> (-273.05, -209.55) projected
  arc A1 (-209.55, -273.05) -> (-273.05, -209.55) centre (-273.05, -273.05) ccw projected
  line L66 (-209.55, -273.05) -> (-209.55, -355.6) projected
  line L67 (-209.55, -355.6) -> (-177.8, -355.6) projected
  line L68 (-177.8, -355.6) -> (-177.8, -323.85) projected
  line L69 (-177.8, -323.85) -> (-146.05, -323.85) projected
  line L70 (-146.05, -323.85) -> (-146.05, -279.4) projected
  line L71 (-146.05, -279.4) -> (-107.95, -279.4) projected
  line L72 (-107.95, -279.4) -> (-107.95, -323.85) projected
  line L73 (-107.95, -323.85) -> (-76.2, -323.85) projected
  line L74 (-76.2, -323.85) -> (-76.2, -355.6) projected
  line L75 (-76.2, -355.6) -> (-50.8, -355.6) projected
  line L76 (-50.8, -355.6) -> (-50.8, -323.85) projected
  line L77 (-50.8, -323.85) -> (-19.05, -323.85) projected
  line L78 (-19.05, -323.85) -> (-19.05, -279.4) projected
  line L79 (-19.05, -279.4) -> (19.05, -279.4) projected
  line L80 (19.05, -279.4) -> (19.05, -323.85) projected
  line L81 (19.05, -323.85) -> (50.8, -323.85) projected
  line L82 (50.8, -323.85) -> (50.8, -355.6) projected
  line L83 (50.8, -355.6) -> (79.9338, -355.6) projected
  line L84 (79.9338, -355.6) -> (79.9338, -323.85) projected
  line L85 (79.9338, -323.85) -> (101.4222, -323.85) projected
  line L86 (101.4222, -323.85) -> (104.0638, -321.2084) projected
  line L87 (104.0638, -321.2084) -> (104.0638, -283.1084) projected
  line L88 (104.0638, -283.1084) -> (114.1222, -273.05) projected
  line L89 (114.1222, -273.05) -> (157.48, -273.05) projected
  line L90 (157.48, -273.05) -> (167.5384, -283.1084) projected
  line L91 (167.5384, -283.1084) -> (167.5384, -321.2084) projected
  line L92 (167.5384, -321.2084) -> (170.18, -323.85) projected
  line L93 (170.18, -323.85) -> (196.85, -323.85) projected
  line L94 (196.85, -323.85) -> (196.85, -355.6) projected
  line L95 (196.85, -355.6) -> (209.55, -355.6) projected
  line L96 (209.55, -355.6) -> (209.55, -273.05) projected
  arc A2 (273.05, -209.55) -> (209.55, -273.05) centre (273.05, -273.05) ccw projected
  line L97 (273.05, -209.55) -> (355.6, -209.55) projected
  line L98 (355.6, -209.55) -> (355.6, 209.55) projected
  line L99 (355.6, 209.55) -> (273.05, 209.55) projected
  arc A3 (209.55, 273.05) -> (273.05, 209.55) centre (273.05, 273.05) ccw projected
  line L100 (209.55, 273.05) -> (209.55, 355.6) projected
  line L101 (209.55, 355.6) -> (196.85, 355.6) projected
  line L102 (196.85, 355.6) -> (196.85, 323.85) projected
  line L103 (196.85, 323.85) -> (170.18, 323.85) projected
  line L104 (170.18, 323.85) -> (167.5384, 321.2084) projected
  line L105 (167.5384, 321.2084) -> (167.5384, 283.1084) projected
  line L106 (167.5384, 283.1084) -> (157.48, 273.05) projected
  line L107 (157.48, 273.05) -> (114.1222, 273.05) projected
  line L108 (114.1222, 273.05) -> (104.0638, 283.1084) projected
  line L109 (104.0638, 283.1084) -> (104.0638, 321.2084) projected
  line L110 (104.0638, 321.2084) -> (101.4222, 323.85) projected
  line L111 (101.4222, 323.85) -> (79.9338, 323.85) projected
  line L112 (79.9338, 323.85) -> (79.9338, 355.6) projected
  line L113 (79.9338, 355.6) -> (50.8, 355.6) projected
  line L114 (50.8, 355.6) -> (50.8, 323.85) projected
  line L115 (50.8, 323.85) -> (19.05, 323.85) projected
  line L116 (19.05, 323.85) -> (19.05, 279.4) projected
  line L117 (19.05, 279.4) -> (-19.05, 279.4) projected
  line L118 (-19.05, 279.4) -> (-19.05, 323.85) projected
  line L119 (-19.05, 323.85) -> (-50.8, 323.85) projected
  line L120 (-50.8, 323.85) -> (-50.8, 355.6) projected
  line L121 (-50.8, 355.6) -> (-76.2, 355.6) projected
  line L122 (-76.2, 355.6) -> (-76.2, 323.85) projected
  line L123 (-76.2, 323.85) -> (-107.95, 323.85) projected
  line L124 (-107.95, 323.85) -> (-107.95, 279.4) projected
  line L125 (-107.95, 279.4) -> (-146.05, 279.4) projected
  line L126 (-146.05, 279.4) -> (-146.05, 323.85) projected
  line L127 (-146.05, 323.85) -> (-177.8, 323.85) projected
  line L128 (44.45, 120.65) -> (-177.8, 120.65)
  line L129 (-177.8, 120.65) -> (-177.8, 127)
  line L130 (44.45, -120.65) -> (-177.8, -120.65)
  line L131 (-177.8, -120.65) -> (-177.8, -127)
  line L132 (-76.2, 127) -> (-50.8, 127)
  line L133 (-76.2, -127) -> (-50.8, -127)
  point P0 (0, 0)
  constraints: 12 end point, 3 perpendicular, 2 collinear, 1 parallel, 1 point on line
extrude "Extrusion8" cut sketch "Sketch8" against normal blind 25.4 contours L133 L17 L131 L130 L7 L6 | L132 L38 L37 L128 L129 L24
sketch "Sketch9" plane through (0, 6.35, 0) normal (0, 1, 0) x (1, 0, 0)
  line L0 (0, -395.3537) -> (0, 422.9924)
  line L1 (-177.8, 323.85) -> (-177.8, 355.6) projected
  line L2 (-177.8, 355.6) -> (-209.55, 355.6) projected
  line L3 (-209.55, 355.6) -> (-209.55, 273.05) projected
  arc A0 (-273.05, 209.55) -> (-209.55, 273.05) centre (-273.05, 273.05) ccw projected
  line L4 (-273.05, 209.55) -> (-355.6, 209.55) projected
  line L5 (-355.6, 209.55) -> (-355.6, 190.5) projected
  line L6 (-355.6, 190.5) -> (-323.85, 190.5) projected
  line L7 (-323.85, 190.5) -> (-323.85, 158.75) projected
  line L8 (-323.85, 158.75) -> (-279.4, 158.75) projected
  line L9 (-279.4, 158.75) -> (-279.4, 120.65) projected
  line L10 (-279.4, 120.65) -> (-323.85, 120.65) projected
  line L11 (-323.85, 120.65) -> (-323.85, 88.9) projected
  line L12 (-323.85, 88.9) -> (-355.6, 88.9) projected
  line L13 (-355.6, 88.9) -> (-355.6, -88.9) projected
  line L14 (-355.6, -88.9) -> (-323.85, -88.9) projected
  line L15 (-323.85, -88.9) -> (-323.85, -120.65) projected
  line L16 (-323.85, -120.65) -> (-279.4, -120.65) projected
  line L17 (-279.4, -120.65) -> (-279.4, -158.75) projected
  line L18 (-279.4, -158.75) -> (-323.85, -158.75) projected
  line L19 (-323.85, -158.75) -> (-323.85, -190.5) projected
  line L20 (-323.85, -190.5) -> (-355.6, -190.5) projected
  line L21 (-355.6, -190.5) -> (-355.6, -209.55) projected
  line L22 (-355.6, -209.55) -> (-273.05, -209.55) projected
  arc A1 (-209.55, -273.05) -> (-273.05, -209.55) centre (-273.05, -273.05) ccw projected
  line L23 (-209.55, -273.05) -> (-209.55, -355.6) projected
  line L24 (-209.55, -355.6) -> (-177.8, -355.6) projected
  line L25 (-177.8, -355.6) -> (-177.8, -323.85) projected
  line L26 (-177.8, -323.85) -> (-146.05, -323.85) projected
  line L27 (-146.05, -323.85) -> (-146.05, -279.4) projected
  line L28 (-146.05, -279.4) -> (-107.95, -279.4) projected
  line L29 (-107.95, -279.4) -> (-107.95, -323.85) projected
  line L30 (-107.95, -323.85) -> (-76.2, -323.85) projected
  line L31 (-76.2, -323.85) -> (-76.2, -355.6) projected
  line L32 (-76.2, -355.6) -> (-50.8, -355.6) projected
  line L33 (-50.8, -355.6) -> (-50.8, -323.85) projected
  line L34 (-50.8, -323.85) -> (-19.05, -323.85) projected
  line L35 (-19.05, -323.85) -> (-19.05, -279.4) projected
  line L36 (-19.05, -279.4) -> (19.05, -279.4) projected
  line L37 (19.05, -279.4) -> (19.05, -323.85) projected
  line L38 (19.05, -323.85) -> (50.8, -323.85) projected
  line L39 (50.8, -323.85) -> (50.8, -355.6) projected
  line L40 (50.8, -355.6) -> (79.9338, -355.6) projected
  line L41 (79.9338, -355.6) -> (79.9338, -323.85) projected
  line L42 (79.9338, -323.85) -> (101.4222, -323.85) projected
  line L43 (101.4222, -323.85) -> (104.0638, -321.2084) projected
  line L44 (104.0638, -321.2084) -> (104.0638, -283.1084) projected
  line L45 (104.0638, -283.1084) -> (114.1222, -273.05) projected
  line L46 (114.1222, -273.05) -> (157.48, -273.05) projected
  line L47 (157.48, -273.05) -> (167.5384, -283.1084) projected
  line L48 (167.5384, -283.1084) -> (167.5384, -321.2084) projected
  line L49 (167.5384, -321.2084) -> (170.18, -323.85) projected
  line L50 (170.18, -323.85) -> (196.85, -323.85) projected
  line L51 (196.85, -323.85) -> (196.85, -355.6) projected
  line L52 (196.85, -355.6) -> (209.55, -355.6) projected
  line L53 (209.55, -355.6) -> (209.55, -273.05) projected
  arc A2 (273.05, -209.55) -> (209.55, -273.05) centre (273.05, -273.05) ccw projected
  line L54 (273.05, -209.55) -> (355.6, -209.55) projected
  line L55 (355.6, -209.55) -> (355.6, 209.55) projected
  line L56 (355.6, 209.55) -> (273.05, 209.55) projected
  arc A3 (209.55, 273.05) -> (273.05, 209.55) centre (273.05, 273.05) ccw projected
  line L57 (209.55, 273.05) -> (209.55, 355.6) projected
  line L58 (209.55, 355.6) -> (196.85, 355.6) projected
  line L59 (196.85, 355.6) -> (196.85, 323.85) projected
  line L60 (196.85, 323.85) -> (170.18, 323.85) projected
  line L61 (170.18, 323.85) -> (167.5384, 321.2084) projected
  line L62 (167.5384, 321.2084) -> (167.5384, 283.1084) projected
  line L63 (167.5384, 283.1084) -> (157.48, 273.05) projected
  line L64 (157.48, 273.05) -> (114.1222, 273.05) projected
  line L65 (114.1222, 273.05) -> (104.0638, 283.1084) projected
  line L66 (104.0638, 283.1084) -> (104.0638, 321.2084) projected
  line L67 (104.0638, 321.2084) -> (101.4222, 323.85) projected
  line L68 (101.4222, 323.85) -> (79.9338, 323.85) projected
  line L69 (79.9338, 323.85) -> (79.9338, 355.6) projected
  line L70 (79.9338, 355.6) -> (50.8, 355.6) projected
  line L71 (50.8, 355.6) -> (50.8, 323.85) projected
  line L72 (50.8, 323.85) -> (19.05, 323.85) projected
  line L73 (19.05, 323.85) -> (19.05, 279.4) projected
  line L74 (19.05, 279.4) -> (-19.05, 279.4) projected
  line L75 (-19.05, 279.4) -> (-19.05, 323.85) projected
  line L76 (-19.05, 323.85) -> (-50.8, 323.85) projected
  line L77 (-50.8, 323.85) -> (-50.8, 355.6) projected
  line L78 (-50.8, 355.6) -> (-76.2, 355.6) projected
  line L79 (-76.2, 355.6) -> (-76.2, 323.85) projected
  line L80 (-76.2, 323.85) -> (-107.95, 323.85) projected
  line L81 (-107.95, 323.85) -> (-107.95, 279.4) projected
  line L82 (-107.95, 279.4) -> (-146.05, 279.4) projected
  line L83 (-146.05, 279.4) -> (-146.05, 323.85) projected
  line L84 (-146.05, 323.85) -> (-177.8, 323.85) projected
  line L85 (-50.8, -127) -> (-76.2, -127) projected
  line L86 (-76.2, -127) -> (-76.2, -158.75) projected
  line L87 (-76.2, -158.75) -> (-107.95, -158.75) projected
  line L88 (-107.95, -158.75) -> (-107.95, -203.2) projected
  line L89 (-107.95, -203.2) -> (-146.05, -203.2) projected
  line L90 (-146.05, -203.2) -> (-146.05, -158.75) projected
  line L91 (-146.05, -158.75) -> (-177.8, -158.75) projected
  line L92 (-177.8, -158.75) -> (-177.8, -120.65) projected
  line L93 (-177.8, -120.65) -> (101.6, -120.65) projected
  line L94 (101.6, -120.65) -> (101.6, -82.55) projected
  line L95 (101.6, -82.55) -> (142.1384, -82.55) projected
  line L96 (142.1384, -82.55) -> (142.1384, -196.85) projected
  line L97 (142.1384, -196.85) -> (101.6, -196.85) projected
  line L98 (101.6, -196.85) -> (101.6, -158.75) projected
  line L99 (101.6, -158.75) -> (19.05, -158.75) projected
  line L100 (19.05, -158.75) -> (19.05, -203.2) projected
  line L101 (19.05, -203.2) -> (-19.05, -203.2) projected
  line L102 (-19.05, -203.2) -> (-19.05, -158.75) projected
  line L103 (-19.05, -158.75) -> (-50.8, -158.75) projected
  line L104 (-50.8, -158.75) -> (-50.8, -127) projected
  line L105 (-177.8, 120.65) -> (-177.8, 158.75) projected
  line L106 (-177.8, 158.75) -> (-146.05, 158.75) projected
  line L107 (-146.05, 158.75) -> (-146.05, 203.2) projected
  line L108 (-146.05, 203.2) -> (-107.95, 203.2) projected
  line L109 (-107.95, 203.2) -> (-107.95, 158.75) projected
  line L110 (-107.95, 158.75) -> (-76.2, 158.75) projected
  line L111 (-76.2, 158.75) -> (-76.2, 127) projected
  line L112 (-76.2, 127) -> (-50.8, 127) projected
  line L113 (-50.8, 127) -> (-50.8, 158.75) projected
  line L114 (-50.8, 158.75) -> (-19.05, 158.75) projected
  line L115 (-19.05, 158.75) -> (-19.05, 203.2) projected
  line L116 (-19.05, 203.2) -> (19.05, 203.2) projected
  line L117 (19.05, 203.2) -> (19.05, 158.75) projected
  line L118 (19.05, 158.75) -> (101.6, 158.75) projected
  line L119 (101.6, 158.75) -> (101.6, 196.85) projected
  line L120 (101.6, 196.85) -> (142.1384, 196.85) projected
  line L121 (142.1384, 196.85) -> (142.1384, 82.55) projected
  line L122 (142.1384, 82.55) -> (101.6, 82.55) projected
  line L123 (101.6, 82.55) -> (101.6, 120.65) projected
  line L124 (101.6, 120.65) -> (-177.8, 120.65) projected
  point P0 (0, 0)
  point P1 (0, 279.4)
  point P2 (0, 203.2)
  point P3 (0, 120.65)
  point P4 (0, -120.65)
  point P5 (0, -203.2)
  point P6 (0, -279.4)
  constraints: 2 end point, 1 vertical
extrude "Extrusion9" cut sketch "Sketch9" against normal blind 23.8125 contours L0 L101 L100 L99 L98 L97 L96 L95 L94 L93 L124 L123 L122 L121 L120 L119 L118 L117 L116 L74 L73 L72 L71 L70 L69 L68 L67 L66 L65 L64 L63 L62 L61 L60 L59 L58 L57 A3 L56 L55 L54 A2 L53 L52 L51 L50 L49 L48 L47 L46 L45 L44 L43 L42 L41 L40 L39 L38 L37 L36
body "Solid1"
